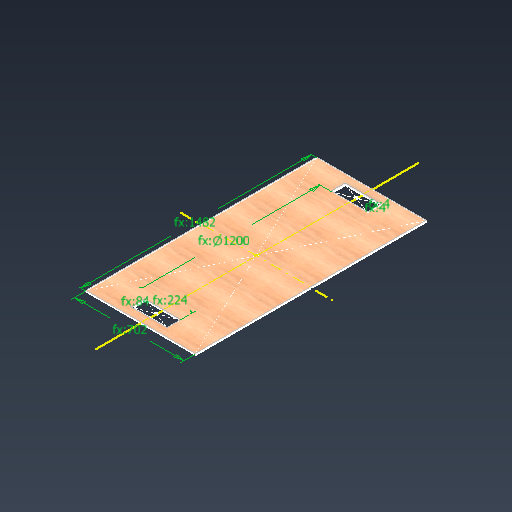
# Autodesk Inventor part: GroundPlate
Saved by Autodesk Inventor 2021.4 (Build 254397000, 397)
## iProperties
Created: 2021-11-23
Part Number: GroundPlate
Material: Generic
Document SubType Name: Modeling
Designer: jo_ki
Density: 1 g/cm^3
Appearance: Birch - Natural Polished
Author: jo_ki
Autodesk Inventor part; units mm, degrees
ref_plane "YZ Plane" through (0, 0, 0) normal (1, 0, 0) x (0, 1, 0)
ref_plane "XZ Plane" through (0, 0, 0) normal (0, 1, 0) x (-1, 0, 0)
ref_plane "XY Plane" through (0, 0, 0) normal (0, 0, 1) x (1, 0, 0)
derived "Mastersketch.ipt"
sketch "Sketch1" plane through (0, 0, 0) normal (0, 1, 0) x (-1, 0, 0)
  line L0 (-351, 741) -> (351, 741)
  line L1 (351, 741) -> (351, -741)
  line L2 (351, -741) -> (-351, -741)
  line L3 (-351, -741) -> (-351, 741)
  line L4 (-351, 741) -> (351, -741) construction
  line L5 (351, 741) -> (-351, -741) construction
  line L6 (-112, 684) -> (112, 684)
  line L7 (112, 684) -> (112, 600)
  line L8 (112, 600) -> (-112, 600)
  line L9 (-112, 600) -> (-112, 684)
  line L10 (-112, 684) -> (112, 600) construction
  line L11 (112, 684) -> (-112, 600) construction
  line L12 (-112, -684) -> (112, -684)
  line L13 (112, -684) -> (112, -600)
  line L14 (112, -600) -> (-112, -600)
  line L15 (-112, -600) -> (-112, -684)
  line L16 (-112, -684) -> (112, -600) construction
  line L17 (112, -684) -> (-112, -600) construction
  line L18 (0, -1037.4) -> (0, 1037.4) projected
  line L19 (491.4, 0) -> (-491.4, 0) projected
  line L20 (116, -688) -> (-116, -688)
  line L21 (-116, -688) -> (-116, -600)
  line L22 (-116, -600) -> (116, -600)
  line L23 (116, -600) -> (116, -688)
  line L24 (116, -688) -> (-116, -600) construction
  line L25 (-116, -688) -> (116, -600) construction
  point P0 (0, 0)
  point P1 (0, 642)
  point P2 (0, -642)
  point P3 (0, 642)
  point P4 (0, -642)
  point P5 (0, -644)
  dimension "d1" = 1482
  dimension "d2" = 702
  dimension "d3" = 224
  dimension "d4" = 84
  dimension "d5" = 1200
  dimension "d8" = 4
  dimension "d9" = 4
  constraints: 48 end point, 10 midpoint, 8 parallel, 4 horizontal, 4 perpendicular, 3 point on line, 2 equal length, 1 collinear, 1 symmetric about line
  measures "d1" distance of L0.end L1.end
  measures "d2" distance of L0.start L0.end
  measures "d3" distance of L7.end L8.end
  measures "d4" distance of L6.end L7.end
  measures "d5" diameter of L8 L19
  measures "d8" distance between parallel lines of L21 L15
  measures "d9" distance between parallel lines of L20 L12
extrude "Extrusion1" add sketch "Sketch1" along normal mid plane 8
extrude "Extrusion2" cut sketch "Sketch1" along normal through all both and the other way through all contours L18 L12 L15 L14 | L14 L13 L12 L18 | L20 L21 L22 L15 L12 L18 | L18 L12 L13 L22 L23 L20
mirror "Mirror1" about plane through (0, 0, 0) normal (0, 0, 1) of "Extrusion2"
equation "\"d1\" = groundPlate_length"
equation "\"d2\" = groundPlate_width"
equation "\"d3\" = goal_width"
equation "\"d4\" = goal_depth"
equation "\"d5\" = glass_length"
equation "\"d8\" = goalPanel_thickness"
equation "\"d9\" = goalPanel_thickness"
equation "\"d6\" = groundPlate_thickness"
equation "\"groundPlate_length\" = 1482"
equation "\"groundPlate_width\" = 702"
equation "\"goal_width\" = 224"
equation "\"goal_depth\" = 84"
equation "\"glass_length\" = 1200"
equation "\"goalPanel_thickness\" = 4"
equation "\"groundPlate_thickness\" = 8"
body "Solid1"
